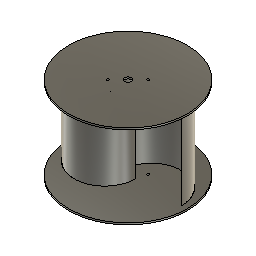
Savonius Turbine (Autodesk Fusion 360 design; units mm, degrees)
Autodesk Fusion 360 part; units mm, degrees
note: some values were not read from the file. Set by a fixed rule: which face or edge a step refers to.
sketch "Turbine Blade" plane through (0, 0, 0) normal (0, 0, 1) x (1, 0, 0) in component "Savonius Turbine"
  circle A0 centre (0, 0) radius 10.5 construction
  line L0 (0, 0) -> (-10.5, 0) construction
  line L1 (-10.5, 0) -> (75, 0) construction
  arc A1 (75, 0) -> (-10.5, 0) centre (32.25, 0) ccw
  arc A2 (74.2, 0) -> (-9.7, 0) centre (32.25, 0) ccw
  line L2 (74.2, 0) -> (75, 0)
  line L3 (-10.5, 0) -> (-9.7, 0) construction
  line L4 (-9.7, 0) -> (-10.5, 0)
  dimension "d57" = 21
  dimension "d59" = 75
  constraint coincident A0.centre L0.start
  constraint coincident A0 L0.end
  constraint horizontal L0
  constraint horizontal L1
  constraint parallel L1 L2
  constraint parallel L1 L3
  measures "d57" diameter of A0
  measures "d59" distance of L1.end A0.centre
extrude "Extrude5" add sketch "Turbine Blade" along normal blind 115.5 makes body 1 in component "Savonius Turbine"
pattern_circular "C-Pattern1" count 2 over 360 about axis through (0, 0, 1.75) along (0, 0, 1) of bodies 1 makes body 2 in component "Savonius Turbine"
sketch "EndPlates" plane through (0, 0, 0) normal (0, 0, 1) x (1, 0, 0) in component "Savonius Turbine"
  circle A0 centre (0, 0) radius 82.5
  line L0 (14.1421, 14.1421) -> (-14.1421, -14.1421) construction
  circle A1 centre (14.1421, 14.1421) radius 1.5
  circle A2 centre (-14.1421, -14.1421) radius 1.5
  line L1 (20, 0) -> (2.5, 0)
  circle A3 centre (0, 0) radius 4.5
  dimension "d65" = 165
  dimension "d68" = 40
  dimension "d69" = 3
  dimension "d70" = 3
  dimension "d71" = 45
  dimension "d72" = 9
  constraint coincident A0.centre A3.centre
  constraint midpoint L0 A0.centre
  constraint coincident L0.start A1.centre
  constraint coincident L0.end A2.centre
  constraint concentric A0 A3
  measures "d65" diameter of A0
  measures "d68" distance of L0.start L0.end
  measures "d69" diameter of A1
  measures "d70" diameter of A2
  measures "d71" angle of L0 L1
  measures "d72" diameter of A3
extrude "Extrude6" add sketch "EndPlates" along normal blind 2.4 separate body makes body 3 in component "Savonius Turbine"
extrude "Extrude7" add sketch "EndPlates" along normal mid plane 2.4 from surface at 115.5 separate body makes body 4 in component "Savonius Turbine"
combine "Combine1" operation cut target body 4 tool bodies 1 2 keep tools in component "Savonius Turbine"
combine "Combine2" operation add target body 3 tool bodies 2 1 in component "Savonius Turbine"
move_face "OffsetFaces1" offset -0.1 8 faces at (73.9915, 4.1769, 114.7) (-73.9915, -4.1769, 114.7) (-9.9667, 0, 114.7) (74.7876, 4.2565, 114.7) (9.9667, 0, 114.7) (-74.7876, -4.2565, 114.7) (74.4667, 0, 114.7) (-74.4667, 0, 114.7) on bodies 4 in component "Savonius Turbine"
component "Savonius Turbine" placed x (1, 0, 0) y (0, 1, 0) z (0, 0, 1) at (0, 0, 0)
equation "Width = 150 mm" comment "Width of the turbine"
equation "AspectRatio = 0.77"
equation "OverlapPercent = 0.14" comment "How far the blades should overlap.  e.g. 0.10 would be 10%"
equation "Height = Width * AspectRatio"
equation "Overlap = OverlapPercent * Width"
equation "BladeDiameter = ( Width + Overlap ) / 2"
equation "BladeThickness = 0.8 mm"
equation "BaseThickness = 2.4 mm"
equation "Twist = 0.5"
equation "NumberOfBlades = 2"
equation "d57 = Overlap"
equation "d59 = Width / 2"
equation "d60 = -BladeThickness"
equation "d61 = Height"
equation "d63 = NumberOfBlades"
equation "d65 = Width * BaseRatio"
equation "d66 = BaseThickness"
equation "d73 = Height"
equation "d74 = BaseThickness"
equation "BaseRatio = 1.1" comment "This is the ratio of the diameter of the end plates to the width.  e.g. 1.1 means the end plates are 10% larger than the width"
named bodies: "Blade1", "Blade2", "Top", "Bottom"
